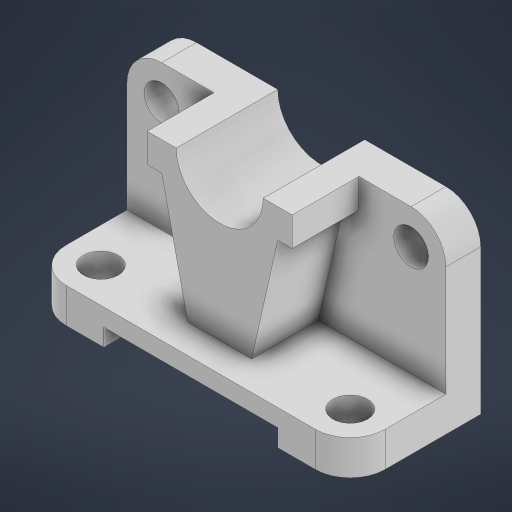
# Autodesk Inventor part: Część8
Saved by Autodesk Inventor 2023 (Build 270158000, 158)
## iProperties
Created: 2023-05-07
Part Number: Część8
Material: Ogólny
Document SubType Name: Modeling
Designer: Adam
Density: 1 g/cm^3
Appearance: Domyślna
Author: Adam
Autodesk Inventor part; units mm, degrees
ref_plane "YZ Plane" through (0, 0, 0) normal (1, 0, 0) x (0, 1, 0)
ref_plane "XZ Plane" through (0, 0, 0) normal (0, 1, 0) x (-1, 0, 0)
ref_plane "XY Plane" through (0, 0, 0) normal (0, 0, 1) x (1, 0, 0)
sketch "Szkic1" plane through (0, 0, 0) normal (0, 1, 0) x (-1, 0, 0)
  line L0 (55, -12.5) -> (-55, -12.5)
  line L1 (-55, -12.5) -> (-55, 20.5)
  line L2 (-43, 32.5) -> (43, 32.5)
  line L3 (55, 20.5) -> (55, -12.5)
  arc A0 (55, 20.5) -> (43, 32.5) centre (43, 20.5) ccw
  arc A1 (-43, 32.5) -> (-55, 20.5) centre (-43, 20.5) ccw
  point P0 (0, 0)
  point P1 (-55, 32.5)
  point P2 (55, 32.5)
  dimension "d0" = 110
  dimension "d1" = 45
  dimension "d2" = 12
  constraints: 8 end point, 4 point on circle, 4 point on line, 4 tangent, 2 centre point, 2 parallel, 1 equal radius, 1 horizontal, 1 perpendicular
  measures "d0" distance of point (-55, 32.5) point (55, 32.5)
  measures "d1" distance of L0.end point (-55, 32.5)
  measures "d2" radius of A0
extrude "Wyciągnięcie proste1" add sketch "Szkic1" along normal blind 12
sketch "Szkic2" plane through (0, 12, 0) normal (0, 1, 0) x (1, 0, 0)
  line L0 (55, 12.5) -> (-55, 12.5) projected
  line L1 (-55, 12.5) -> (55, 12.5)
  line L2 (55, 12.5) -> (55, 0.5)
  line L3 (55, 0.5) -> (-55, 0.5)
  line L4 (-55, 0.5) -> (-55, 12.5)
  point P0 (0, 0)
  dimension "d5" = 12
  constraints: 8 end point, 2 parallel, 1 horizontal, 1 perpendicular
  measures "d5" distance of L1.end L2.end
extrude "Wyciągnięcie proste2" add sketch "Szkic2" along normal blind 50
fillet "Zaokrąglenie1" radius 12 2 edges at (55, 62, -6.5) (-55, 62, -6.5)
sketch "Szkic3" plane through (-55, 12, -0.5) normal (0, 0, 1) x (1, 0, 0)
  line L0 (98, 50) -> (12, 50) projected
  line L1 (30, 50) -> (80, 50)
  line L2 (80, 50) -> (80, 40)
  line L3 (80, 40) -> (30, 40)
  line L4 (30, 40) -> (30, 50)
  line L5 (0, 0) -> (0, 38) projected
  line L6 (35, 40) -> (44, 0)
  line L7 (110, 0) -> (0, 0) projected
  line L8 (75, 40) -> (66, 0)
  line L9 (44, 0) -> (66, 0)
  line L10 (44, 0) -> (66, 0)
  line L11 (110, 0) -> (110, 38) projected
  point P0 (55, -12)
  point P1 (66, 0)
  dimension "d9" = 50
  dimension "d10" = 30
  dimension "d11" = 10
  dimension "d12" = 44
  dimension "d13" = 44
  constraints: 16 end point, 4 point on line, 2 collinear, 2 parallel, 1 horizontal, 1 perpendicular
  measures "d9" distance between parallel lines of L2 L4
  measures "d10" distance between parallel lines of L5 L4
  measures "d11" distance between parallel lines of L3 L0
  measures "d12" distance from line of L11 L8.end
  measures "d13" distance from line of L5 L6.end
extrude "Wyciągnięcie proste3" add sketch "Szkic3" along normal blind 23
sketch "Szkic4" plane through (-55, 12, 22.5) normal (0, 0, 1) x (1, 0, 0)
  line L0 (98, 50) -> (12, 50) projected
  point P0 (55, -12)
  point P1 (55, 50)
  constraints: 1 midpoint
hole "Otwór1" at (0, 62, 22.5) direction (0, 0, -1) diameter 30 end through all
sketch "Szkic5" plane through (-55, 12, -0.5) normal (0, 0, 1) x (1, 0, 0)
  arc A0 (12, 50) -> (0, 38) centre (12, 38) ccw projected
  arc A1 (110, 38) -> (98, 50) centre (98, 38) ccw projected
  point P0 (55, -12)
  constraints: 2 coincident
hole "Otwór2" at (-43, 50, -0.5) at (43, 50, -0.5) direction (0, 0, -1) diameter 12 end through all
sketch "Szkic6" plane through (0, 12, 0) normal (0, 1, 0) x (1, 0, 0)
  arc A0 (-55, -20.5) -> (-43, -32.5) centre (-43, -20.5) ccw projected
  arc A1 (43, -32.5) -> (55, -20.5) centre (43, -20.5) ccw projected
  point P0 (0, 0)
  constraints: 2 coincident
hole "Otwór3" at (-43, 12, 20.5) at (43, 12, 20.5) direction (0, -1, 0) diameter 12 end through all
sketch "Szkic7" plane through (0, 0, 0) normal (0, -1, 0) x (1, 0, 0)
  line L0 (-43, 32.5) -> (43, 32.5) projected
  line L1 (-30, 32.5) -> (30, 32.5)
  line L2 (30, 32.5) -> (30, 0)
  line L3 (30, 0) -> (-30, 0)
  line L4 (-30, 0) -> (-30, 32.5)
  point P0 (0, 0)
  dimension "d37" = 60
  constraints: 8 end point, 2 parallel, 1 horizontal, 1 perpendicular, 1 point on line
  measures "d37" distance of L2.end L3.end
extrude "Wyciągnięcie proste4" cut sketch "Szkic7" against normal blind 6
